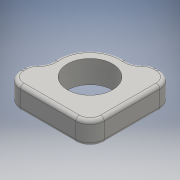
# Autodesk Inventor part: polaris_K05_front
Saved by Autodesk Inventor 2016 (Build 200138000, 138)
## iProperties
Created: 2015-09-04
Part Number: polaris_K05_front
Material: Generic
Document SubType Name: Modeling
Designer: HE BEC
Density: 1 g/cm^3
Appearance: Default
Author: HE BEC
Autodesk Inventor part; units mm, degrees
ref_plane "YZ Plane" through (0, 0, 0) normal (1, 0, 0) x (0, 1, 0)
ref_plane "XZ Plane" through (0, 0, 0) normal (0, 1, 0) x (-1, 0, 0)
ref_plane "XY Plane" through (0, 0, 0) normal (0, 0, 1) x (1, 0, 0)
sketch "Sketch1" plane through (0, 0, 0) normal (0, 0, 1) x (1, 0, 0)
  line L0 (0, 0) -> (-24.5, 0) construction
  line L1 (-24.5, 0) -> (-24.5, 24.5) construction
  line L2 (-24.5, 24.5) -> (0, 24.5) construction
  line L3 (0, 24.5) -> (0, 0) construction
  line L4 (-0.9, 0.9) -> (-24.5, 0.9)
  line L5 (-24.5, 0.9) -> (-24.5, 24.5)
  line L6 (-24.5, 24.5) -> (-0.9, 24.5)
  line L7 (-0.9, 24.5) -> (-0.9, 0.9)
  circle A0 centre (-12.7, 12.7) radius 6.35
  line L8 (0, 25.4) -> (-29.8306, 25.4) construction
  line L9 (-25.4, 0) -> (-25.4, 30.1539) construction
  point P0 (-3.5, 21.9)
  point P1 (-3.5, 3.5)
  point P2 (-21.9, 3.5)
  dimension "d0" = 24.5
  dimension "d3" = 0.9
  dimension "d4" = 12.7
  dimension "d5" = 12.7
  dimension "d6" = 12.7
  dimension "d7" = 3.5
  dimension "d9" = 25.4
  dimension "d10" = 3.5
  dimension "d11" = 3.5
  dimension "d12" = 25.4
  dimension "d13" = 3.5
  constraints: 20 end point, 4 parallel, 4 perpendicular, 3 horizontal, 1 centre point, 1 horizontal alignment, 1 vertical, 1 vertical alignment
  measures "d0" distance of L2.end L0.start
  measures "d3" distance between parallel lines of L3 L7
  measures "d4" diameter of A0
  measures "d5" distance from line of L3 A0.centre
  measures "d6" distance from line of L0 A0.centre
  measures "d7" distance from line of L3 point (-3.5, 21.9)
  measures "d9" distance between parallel lines of L0 L8
  measures "d10" distance from line of point (-3.5, 21.9) L8
  measures "d11" distance from line of L0 point (-21.9, 3.5)
  measures "d12" distance between parallel lines of L3 L9
  measures "d13" distance from line of point (-21.9, 3.5) L9
extrude "Extrusion1" add sketch "Sketch1" along normal blind 6.4
sketch "Sketch2" plane through (0, 0, 6.4) normal (0, 0, 1) x (1, 0, 0)
  circle A0 centre (-12.7, 12.7) radius 6.35 projected
  arc A1 (-8.2055, 20.8989) -> (-20.8989, 8.2055) centre (-12.7, 12.7) ccw
  line L0 (-24.5, 0.9) -> (-0.9, 0.9) projected
  line L1 (-24.5, 24.5) -> (-24.5, 0.9) projected
  line L2 (-24.5, 7.8123) -> (-24.5, 24.5)
  line L3 (-24.5, 24.5) -> (-7.8123, 24.5)
  arc A2 (-24.5, 7.8123) -> (-20.8989, 8.2055) centre (-24.5, 24.5) ccw
  arc A3 (-8.2055, 20.8989) -> (-7.8123, 24.5) centre (-24.5, 24.5) ccw
  point P0 (0, 0)
  dimension "d14" = 3
  constraints: 6 point on circle, 4 end point, 3 centre point, 2 coincident
  measures "d14" radial gap between concentric circles of A0 A1
extrude "Extrusion2" cut sketch "Sketch2" against normal through all contours A1 A2 L1 L3 A3
fillet "Fillet1" radius 4 7 edges at (-8.2055, 20.8989, 3.2) (-7.8123, 24.5, 3.2) (-0.9, 24.5, 3.2) (-20.8989, 8.2055, 3.2) (-24.5, 7.8123, 3.2) (-24.5, 0.9, 3.2) (-0.9, 0.9, 3.2)
fillet "Fillet2" radius 1 1 edges at (-19.3114, 19.3114, 6.4)
fillet "Fillet3" radius 1 1 edges at (-19.3114, 19.3114, 0)
equation "\"d6\" = d5"
equation "\"d10\" = d7"
equation "\"d11\" = d7"
equation "\"d12\" = d9"
equation "\"d13\" = d7"
body "Solid1"
